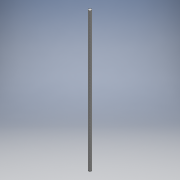
# Autodesk Inventor part: FusoTrapezoidal_8mmx300mm
Saved by Autodesk Inventor 2018 (Build 220112000, 112)
## iProperties
Created: 2018-09-20
Part Number: FusoTrapezoidal_8mmx300mm
Material: Genérico
Document SubType Name: Modeling
Designer: Georgines
Density: 1 g/cm^3
Appearance: Padrão
Author: Georgines
Autodesk Inventor part; units mm, degrees
ref_plane "YZ Plane" through (0, 0, 0) normal (1, 0, 0) x (0, 1, 0)
ref_plane "XZ Plane" through (0, 0, 0) normal (0, 1, 0) x (-1, 0, 0)
ref_plane "XY Plane" through (0, 0, 0) normal (0, 0, 1) x (1, 0, 0)
sketch "Esboço1" plane through (0, 0, 0) normal (0, 0, 1) x (1, 0, 0)
  circle A0 centre (0, 0) radius 4
  dimension "d0" = 8
  constraints: 1 centre point, 1 coincident
  measures "d0" diameter of A0
extrude "Extrusão1" add sketch "Esboço1" along normal blind 400
thread "Rosca1" size "TR8x1.5" class "7e" standard "ISO Metric Trapezoidal Threads" full length
